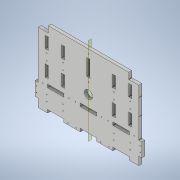
# Autodesk Inventor part: Side_one
Saved by Autodesk Inventor 2020 (Build 240168000, 168)
## iProperties
Created: 2019-12-17
Part Number: Side_one
Material: Generic
Document SubType Name: Modeling
Designer: fabfarm
Density: 1 g/cm^3
Appearance: Default
Author: fabfarm
Autodesk Inventor part; units mm, degrees
ref_plane "YZ Plane" through (0, 0, 0) normal (1, 0, 0) x (0, 1, 0)
ref_plane "XZ Plane" through (0, 0, 0) normal (0, 1, 0) x (-1, 0, 0)
ref_plane "XY Plane" through (0, 0, 0) normal (0, 0, 1) x (1, 0, 0)
sketch "Sketch1" plane through (0, 0, 0) normal (0, 0, 1) x (1, 0, 0)
  line L0 (0, 0) -> (-652, 0)
  line L1 (-652, 0) -> (-652, 464.3)
  line L2 (-652, 464.3) -> (0, 464.3)
  line L3 (0, 464.3) -> (0, 0)
  dimension "d0" = 464.3
  dimension "d1" = 652
  constraints: 8 end point, 2 parallel, 1 horizontal, 1 perpendicular
  measures "d0" distance of L2.end L0.start
  measures "d1" distance of L0.start L0.end
extrude "Extrusion1" add sketch "Sketch1" along normal blind 18.55
sketch "Sketch2" plane through (0, 0, 18.55) normal (0, 0, 1) x (1, 0, 0)
  line L0 (-652, 464.3) -> (-652, 0) projected
  line L1 (-652, 464.3) -> (-633.45, 464.3)
  line L2 (-633.45, 464.3) -> (-633.45, 359.9)
  line L3 (-633.45, 359.9) -> (-652, 359.9)
  line L4 (-652, 359.9) -> (-652, 464.3)
  line L5 (0, 464.3) -> (-652, 464.3) projected
  line L6 (-652, 259.9) -> (-633.45, 259.9)
  line L7 (-633.45, 259.9) -> (-633.45, 134.8)
  line L8 (-633.45, 134.8) -> (-652, 134.8)
  line L9 (-652, 134.8) -> (-652, 259.9)
  point P0 (-652, 359.9)
  point P1 (-652, 134.8)
  dimension "d54" = 18.55
  dimension "d55" = 104.4
  dimension "d86" = 100
  dimension "d87" = 125.1
  constraints: 16 end point, 4 parallel, 2 collinear, 2 horizontal, 2 perpendicular, 2 point on line
  measures "d54" distance of L1.start L1.end
  measures "d55" distance of L1.end L2.end
  measures "d86" distance between parallel lines of L6 L3
  measures "d87" distance of L6.end L7.end
extrude "Extrusion2" cut sketch "Sketch2" against normal blind 18.55
ref_plane "Work Plane1" through (-326, 259.9, 0) normal (-1, 0, 0) x (0, 0, 1)
mirror "Mirror1" about plane through (-326, 259.9, 0) normal (-1, 0, 0) of "Extrusion2"
sketch "Sketch3" plane through (0, 0, 18.55) normal (0, 0, 1) x (1, 0, 0)
  line L0 (0, 464.3) -> (-652, 464.3) projected
  line L1 (-652, 426.35) -> (-572, 426.35)
  line L2 (-572, 426.35) -> (-572, 464.3)
  line L3 (-572, 464.3) -> (-652, 464.3)
  line L4 (-652, 464.3) -> (-652, 426.35)
  point P0 (0, 0)
  point P1 (-18.55, 350)
  dimension "d19" = 80
  dimension "d22" = 37.95
  constraints: 8 end point, 2 perpendicular, 1 parallel, 2 other
  measures "d19" distance of L3.end L2.end
  measures "d22" distance of L3.end L1.start
extrude "Extrusion3" cut sketch "Sketch3" against normal blind 18.55
mirror "Mirror2" about plane through (-326, 259.9, 0) normal (-1, 0, 0) of "Extrusion3"
sketch "Sketch4" plane through (0, 0, 18.55) normal (0, 0, 1) x (1, 0, 0)
  line L0 (-576, 134.8) -> (-476, 134.8)
  line L1 (-476, 134.8) -> (-476, 153.35)
  line L2 (-476, 153.35) -> (-576, 153.35)
  line L3 (-576, 153.35) -> (-576, 134.8)
  line L4 (-376, 134.8) -> (-276, 134.8)
  line L5 (-276, 134.8) -> (-276, 153.35)
  line L6 (-276, 153.35) -> (-376, 153.35)
  line L7 (-376, 153.35) -> (-376, 134.8)
  line L8 (-176, 134.8) -> (-76, 134.8)
  line L9 (-76, 134.8) -> (-76, 153.35)
  line L10 (-76, 153.35) -> (-176, 153.35)
  line L11 (-176, 153.35) -> (-176, 134.8)
  line L12 (0, 0) -> (0, 359.9) projected
  line L13 (-652, 359.9) -> (-652, 0) projected
  line L14 (-633.45, 134.8) -> (-652, 134.8) projected
  line L15 (-652, 259.9) -> (-633.45, 259.9) projected
  dimension "d59" = 100
  dimension "d60" = 100
  dimension "d61" = 100
  dimension "d62" = 100
  dimension "d63" = 100
  dimension "d66" = 18.55
  dimension "d67" = 76
  constraints: 24 end point, 6 parallel, 5 collinear, 3 horizontal, 3 perpendicular
  measures "d59" distance of L1.end L2.end
  measures "d60" distance of L5.end L6.end
  measures "d61" distance between parallel lines of L1 L7
  measures "d62" distance between parallel lines of L11 L5
  measures "d63" distance of L9.end L10.end
  measures "d66" distance of L2.end L0.start
  measures "d67" distance between parallel lines of L12 L9
extrude "Extrusion4" cut sketch "Sketch4" against normal blind 20
sketch "Sketch6" plane through (0, 0, 18.55) normal (0, 0, 1) x (1, 0, 0)
  line L0 (-276, 400.4) -> (-376, 400.4)
  line L1 (-376, 400.4) -> (-376, 425.4)
  line L2 (-376, 425.4) -> (-276, 425.4)
  line L3 (-276, 425.4) -> (-276, 400.4)
  line L4 (-276, 400.4) -> (-376, 425.4) construction
  line L5 (-376, 400.4) -> (-276, 425.4) construction
  line L6 (-326, -92.86) -> (-326, 557.16) projected
  line L7 (-80, 464.3) -> (-572, 464.3) projected
  point P0 (0, 0)
  point P1 (-326, 412.9)
  dimension "d38" = 25
  dimension "d39" = 100
  dimension "d40" = 38.9
  constraints: 12 end point, 2 midpoint, 2 parallel, 1 horizontal, 1 perpendicular, 1 point on line
  measures "d38" distance of L0.end L1.end
  measures "d39" distance of L1.end L2.end
  measures "d40" distance between parallel lines of L7 L2
extrude "Extrusion6" [suppressed]
fillet "Fillet1" [suppressed]
sketch "Sketch7" plane through (0, 0, 18.55) normal (0, 0, 1) x (1, 0, 0)
  line L0 (-590.55, 183.35) -> (-572, 183.35)
  line L1 (-572, 183.35) -> (-572, 253.85)
  line L2 (-572, 253.85) -> (-590.55, 253.85)
  line L3 (-590.55, 253.85) -> (-590.55, 183.35)
  line L4 (-490.6, 183.35) -> (-472.05, 183.35)
  line L5 (-472.05, 183.35) -> (-472.05, 253.85)
  line L6 (-472.05, 253.85) -> (-490.6, 253.85)
  line L7 (-490.6, 253.85) -> (-490.6, 183.35)
  line L8 (-572, 464.3) -> (-572, 426.35) projected
  line L9 (-576, 153.35) -> (-476, 153.35) projected
  point P0 (0, 0)
  point P1 (-572, 290)
  dimension "d44" = 81.4
  dimension "d45" = 18.55
  dimension "d46" = 70.5
  dimension "d72" = 30
  constraints: 16 end point, 4 parallel, 2 collinear, 2 horizontal, 2 perpendicular, 2 point on line
  measures "d44" distance between parallel lines of L7 L1
  measures "d45" distance of L1.end L2.end
  measures "d46" distance of L2.end L0.start
  measures "d72" distance between parallel lines of L9 L0
extrude "Extrusion7" cut sketch "Sketch7" against normal blind 20
mirror "Mirror3" about plane through (-326, 259.9, 0) normal (-1, 0, 0) of "Extrusion7"
sketch "Esquisse8" plane through (0, 0, 0) normal (0, 0, -1) x (-1, 0, 0)
  line L0 (80, 334.35) -> (61.45, 334.35)
  line L1 (61.45, 334.35) -> (61.45, 404.85)
  line L2 (61.45, 404.85) -> (80, 404.85)
  line L3 (80, 404.85) -> (80, 334.35)
  line L4 (161.4, 404.85) -> (179.95, 404.85)
  line L5 (179.95, 404.85) -> (179.95, 334.35)
  line L6 (179.95, 334.35) -> (161.4, 334.35)
  line L7 (161.4, 334.35) -> (161.4, 404.85)
  line L8 (61.45, 183.35) -> (61.45, 253.85) projected
  line L9 (80, 253.85) -> (80, 183.35) projected
  line L10 (161.4, 183.35) -> (161.4, 253.85) projected
  line L11 (179.95, 253.85) -> (179.95, 183.35) projected
  line L12 (80, 253.85) -> (61.45, 253.85) projected
  point P0 (0, 0)
  dimension "d51" = 70.5
  dimension "d90" = 80.5
  constraints: 16 end point, 4 collinear, 4 parallel, 2 horizontal, 2 perpendicular, 2 point on line
  measures "d51" distance of L0.end L1.end
  measures "d90" distance between parallel lines of L0 L12
extrude "Extrusion8" cut sketch "Esquisse8" against normal blind 20
mirror "Symétrie4" about plane through (-326, 259.9, 0) normal (-1, 0, 0) of "Extrusion8"
sketch "Esquisse9" plane through (0, 0, 18.55) normal (0, 0, 1) x (1, 0, 0)
  circle A0 centre (-634.5708, 361.0208) radius 1.585
  circle A1 centre (-634.5708, 135.9208) radius 1.585
  circle A2 centre (-589.4292, 403.7292) radius 1.585
  circle A3 centre (-589.4292, 335.4708) radius 1.585
  circle A4 centre (-634.5708, 258.7792) radius 1.585
  circle A5 centre (-589.4292, 252.7292) radius 1.585
  circle A6 centre (-573.1208, 252.7292) radius 1.585
  circle A7 centre (-573.1208, 184.4708) radius 1.585
  circle A8 centre (-573.1208, 427.4708) radius 1.585
  circle A9 centre (-574.8792, 152.2292) radius 1.585
  circle A10 centre (-374.8792, 152.2292) radius 1.585
  line L0 (-80, 464.3) -> (-572, 464.3) projected
  line L1 (-326, 464.3) -> (-325.9857, 153.4511) construction
  circle A11 centre (-574.8792, 135.9208) radius 1.585
  circle A12 centre (-374.8792, 135.9208) radius 1.585
  line L2 (-633.45, 359.9) -> (-634.5708, 361.0208) construction
  line L3 (-633.45, 426.35) -> (-633.45, 359.9) projected
  line L4 (-633.45, 259.9) -> (-634.5708, 258.7792) construction
  line L5 (-634.5708, 135.9208) -> (-633.45, 134.8) construction
  line L6 (-633.45, 259.9) -> (-633.45, 134.8) projected
  line L7 (-633.45, 426.35) -> (-572, 426.35) projected
  line L8 (-573.1208, 427.4708) -> (-572, 426.35) construction
  line L9 (-590.55, 404.85) -> (-589.4292, 403.7292) construction
  circle A13 centre (-573.1208, 335.4708) radius 1.585
  line L10 (-573.1208, 335.4708) -> (-572, 334.35) construction
  line L11 (-590.55, 334.35) -> (-589.4292, 335.4708) construction
  line L12 (-572, 334.35) -> (-590.55, 334.35) projected
  line L13 (-573.1208, 184.4708) -> (-572, 183.35) construction
  line L14 (-573.1208, 252.7292) -> (-572, 253.85) construction
  line L15 (-572, 253.85) -> (-572, 183.35) projected
  line L16 (-590.55, 183.35) -> (-589.4292, 184.4708) construction
  line L17 (-572, 183.35) -> (-590.55, 183.35) projected
  circle A14 centre (-589.4292, 184.4708) radius 1.585
  line L18 (-572, 334.35) -> (-572, 464.3) projected
  line L19 (-572, 399.325) -> (-490.6, 369.6) construction
  line L20 (-490.6, 334.35) -> (-490.6, 404.85) construction
  line L21 (-531.3, 384.4625) -> (-531.3, 153.45) construction
  circle A15 centre (-473.1708, 403.7292) radius 1.585
  circle A16 centre (-473.1708, 335.4708) radius 1.585
  circle A17 centre (-473.1708, 252.7292) radius 1.585
  circle A18 centre (-489.4792, 252.7292) radius 1.585
  circle A19 centre (-489.4792, 184.4708) radius 1.585
  line L22 (-472.05, 404.85) -> (-473.1708, 403.7292) construction
  circle A20 centre (-489.4792, 335.4708) radius 1.585
  line L23 (-489.4792, 335.4708) -> (-490.6, 334.35) construction
  line L24 (-472.05, 334.35) -> (-473.1708, 335.4708) construction
  line L25 (-489.4792, 184.4708) -> (-490.6, 183.35) construction
  line L26 (-489.4792, 252.7292) -> (-490.6, 253.85) construction
  line L27 (-472.05, 183.35) -> (-473.1708, 184.4708) construction
  circle A21 centre (-473.1708, 184.4708) radius 1.585
  line L28 (-490.6, 334.35) -> (-490.6, 404.85)
  line L29 (-490.6, 399.325) -> (-572, 369.6) construction
  line L30 (-476, 134.8) -> (-576, 134.8) construction
  line L31 (-574.8792, 135.9208) -> (-576, 134.8) construction
  line L32 (-576, 153.35) -> (-476, 153.35) construction
  line L33 (-526, 153.35) -> (-526, 134.8) construction
  circle A22 centre (-477.1208, 152.2292) radius 1.585
  circle A23 centre (-477.1208, 135.9208) radius 1.585
  circle A24 centre (-17.4198, 361.0491) radius 1.585
  circle A25 centre (-17.3991, 135.9491) radius 1.585
  circle A26 centre (-78.9803, 403.6546) radius 1.585
  line L34 (-62.5652, 403.7534) -> (-78.9803, 403.6546) construction
  circle A27 centre (-62.5652, 403.7534) radius 1.585
  circle A28 centre (-62.5589, 335.4949) radius 1.585
  circle A29 centre (-17.4104, 258.8076) radius 1.585
  circle A30 centre (-62.5513, 252.7534) radius 1.585
  circle A31 centre (-78.8598, 252.7519) radius 1.585
  circle A32 centre (-78.8536, 184.4934) radius 1.585
  circle A33 centre (-78.8759, 427.4934) radius 1.585
  circle A34 centre (-77.0921, 152.2521) radius 1.585
  circle A35 centre (-277.0921, 152.2337) radius 1.585
  circle A36 centre (-77.0906, 135.9436) radius 1.585
  circle A37 centre (-277.0906, 135.9253) radius 1.585
  line L35 (-18.5404, 359.9282) -> (-17.4198, 361.0491) construction
  line L36 (-18.5465, 426.3782) -> (-18.5404, 359.9282)
  line L37 (-18.5312, 259.9282) -> (-17.4104, 258.8076) construction
  line L38 (-17.3991, 135.9491) -> (-18.5198, 134.8282) construction
  line L39 (-18.5312, 259.9282) -> (-18.5198, 134.8282)
  line L40 (-18.5465, 426.3782) -> (-79.9965, 426.3726)
  line L41 (-78.8759, 427.4934) -> (-79.9965, 426.3726) construction
  line L42 (-79.9945, 404.8726) -> (-61.4445, 404.8743)
  line L43 (-61.4445, 404.8743) -> (-62.5652, 403.7534) construction
  line L44 (-79.9945, 404.8726) -> (-78.9803, 403.6546) construction
  circle A38 centre (-78.8674, 335.4934) radius 1.585
  line L45 (-78.8674, 335.4934) -> (-79.9881, 334.3726) construction
  line L46 (-61.4381, 334.3743) -> (-62.5589, 335.4949) construction
  line L47 (-79.9881, 334.3726) -> (-61.4381, 334.3743)
  line L48 (-78.8536, 184.4934) -> (-79.9742, 183.3726) construction
  line L49 (-78.8598, 252.7519) -> (-79.9807, 253.8726) construction
  line L50 (-79.9807, 253.8726) -> (-79.9742, 183.3726)
  line L51 (-61.4242, 183.3743) -> (-62.5451, 184.4949) construction
  line L52 (-79.9742, 183.3726) -> (-61.4242, 183.3743)
  circle A39 centre (-62.5451, 184.4949) radius 1.585
  line L53 (-79.9881, 334.3726) -> (-79.9945, 404.8726)
  line L54 (-79.994, 399.3476) -> (-161.3913, 369.6151) construction
  line L55 (-161.3881, 334.3651) -> (-161.3945, 404.8651) construction
  line L56 (-120.6927, 384.4813) -> (-120.6715, 153.4688) construction
  circle A40 centre (-162.5013, 252.7442) radius 1.585
  circle A41 centre (-162.4951, 184.4858) radius 1.585
  circle A42 centre (-162.1087, 403.6455) radius 1.4133
  circle A43 centre (-178.8098, 252.7427) radius 1.585
  line L57 (-162.4951, 184.4858) -> (-161.3742, 183.3651) construction
  line L58 (-162.5013, 252.7442) -> (-161.3807, 253.8651) construction
  line L59 (-179.9242, 183.3634) -> (-178.8036, 184.4843) construction
  circle A44 centre (-178.8036, 184.4843) radius 1.585
  line L60 (-178.8237, 403.7427) -> (-162.1087, 403.6455) construction
  circle A45 centre (-178.8174, 335.4843) radius 1.585
  line L61 (-179.9381, 334.3634) -> (-178.8174, 335.4843) construction
  circle A46 centre (-162.5089, 335.4858) radius 1.585
  line L62 (-161.394, 399.3401) -> (-79.9913, 369.6226) construction
  line L63 (-161.3881, 334.3651) -> (-161.3945, 404.8651)
  line L64 (-162.5089, 335.4858) -> (-161.3881, 334.3651) construction
  circle A47 centre (-178.8237, 403.7427) radius 1.585
  line L65 (-179.9445, 404.8634) -> (-178.8237, 403.7427) construction
  line L66 (-161.3945, 404.8651) -> (-162.1087, 403.6455) construction
  line L67 (-175.9698, 134.8138) -> (-75.9698, 134.8229) construction
  line L68 (-77.0906, 135.9436) -> (-75.9698, 134.8229) construction
  line L69 (-75.9715, 153.3729) -> (-175.9715, 153.3638) construction
  line L70 (-125.9715, 153.3684) -> (-125.9698, 134.8184) construction
  circle A48 centre (-174.8506, 152.2431) radius 1.585
  circle A49 centre (-174.8491, 135.9346) radius 1.585
  line L71 (-590.55, 404.85) -> (-572, 404.85) projected
  circle A50 centre (-573.1208, 403.7292) radius 1.585
  line L72 (-572, 404.85) -> (-573.1208, 403.7292) construction
  circle A51 centre (-489.4792, 403.7292) radius 1.585
  point P0 (-476, 153.35)
  point P1 (-472.05, 183.35)
  point P2 (-276, 153.35)
  point P3 (-472.05, 404.85)
  point P4 (-376, 134.8)
  point P5 (-175.9715, 153.3638)
  point P6 (-179.9242, 183.3634)
  point P7 (-179.9445, 404.8634)
  point P8 (-75.9715, 153.3729)
  point P9 (-275.9698, 134.8046)
  dimension "d69" = 3.17
  dimension "d115" = 45
  dimension "d117" = 45
  dimension "d118" = 45
  dimension "d119" = 45
  dimension "d123" = 45
  dimension "d129" = 45
  dimension "d130" = 45
  dimension "d131" = 45
  dimension "d132" = 45
  dimension "d143" = 45
  dimension "d144" = 45
  constraints: 120 end point, 86 symmetric about line, 14 coincident, 11 centre point, 6 vertical, 5 horizontal alignment, 5 midpoint, 3 vertical alignment, 159 other
  measures "d115" angle of L3 L2
  measures "d117" angle of L6 L5
  measures "d118" angle of L6 L4
  measures "d119" angle of L7 L8
  measures "d123" angle of L12 L11
  measures "d129" angle of L15 L14
  measures "d130" angle of L15 L13
  measures "d131" angle of L17 L16
  measures "d132" angle of L30 L31
  measures "d143" angle of L9 L71
  measures "d144" angle of L18 L72
extrude "Extrusion9" cut sketch "Esquisse9" against normal blind 20
sketch "Esquisse11" plane through (0, 0, 18.55) normal (0, 0, 1) x (1, 0, 0)
  circle A0 centre (-642.725, 329.9) radius 2.25
  circle A1 centre (-642.725, 289.9) radius 2.25
  circle A2 centre (-581.275, 314.35) radius 2.25
  circle A3 centre (-581.275, 273.85) radius 2.25
  circle A4 centre (-481.325, 314.35) radius 2.25
  circle A5 centre (-481.325, 273.85) radius 2.25
  line L0 (-572, 334.35) -> (-590.55, 334.35) projected
  line L1 (-581.275, 334.35) -> (-581.275, 253.85) construction
  line L2 (-590.55, 253.85) -> (-572, 253.85) projected
  line L3 (-472.05, 334.35) -> (-490.6, 334.35) projected
  line L4 (-481.325, 334.35) -> (-481.325, 253.85) construction
  line L5 (-490.6, 253.85) -> (-472.05, 253.85) projected
  line L6 (-633.45, 359.9) -> (-652, 359.9) projected
  line L7 (-80, 464.3) -> (-572, 464.3) projected
  line L8 (-326, 464.3) -> (-326, 153.35) construction
  line L9 (-376, 153.35) -> (-276, 153.35) projected
  circle A6 centre (-9.275, 329.9) radius 2.25
  circle A7 centre (-9.275, 289.9) radius 2.25
  circle A8 centre (-70.725, 314.35) radius 2.25
  circle A9 centre (-70.725, 273.85) radius 2.25
  circle A10 centre (-170.675, 314.35) radius 2.25
  circle A11 centre (-170.675, 273.85) radius 2.25
  line L10 (-70.725, 334.35) -> (-70.725, 253.85) construction
  line L11 (-63.6915, 253.85) -> (-77.7585, 253.85)
  line L12 (-178.265, 334.65) -> (-162.585, 334.65)
  line L13 (-170.675, 334.35) -> (-170.675, 253.85) construction
  line L14 (-162.585, 253.65) -> (-178.265, 253.65)
  line L15 (-16.3085, 359.9) -> (0, 359.9)
  line L16 (-652, 259.9) -> (-633.45, 259.9) projected
  line L17 (-642.725, 359.9) -> (-642.725, 259.9) construction
  point P0 (-573.5723, 199.8)
  point P1 (-588.3085, 334.35)
  point P2 (-588.3085, 253.85)
  point P3 (-574.2415, 253.85)
  point P4 (-473.735, 334.65)
  point P5 (-489.415, 334.65)
  point P6 (-489.415, 253.65)
  point P7 (-473.735, 253.65)
  point P8 (-635.6915, 359.9)
  point P9 (-373.7585, 153.35)
  point P10 (-277.485, 153.35)
  point P11 (-178.265, 253.65)
  point P12 (-635.6915, 259.9)
  point P13 (-490.6, 334.35)
  dimension "d76" = 4.5
  dimension "d79" = 30
  dimension "d80" = 20
  dimension "d81" = 20
  dimension "d82" = 20
  dimension "d83" = 20
  dimension "d91" = 30
  constraints: 18 symmetric about line, 16 end point, 12 centre point, 10 point on line, 5 equal radius, 5 midpoint, 18 other
  measures "d76" diameter of A0
  measures "d79" distance from line of L6 A0.centre
  measures "d80" distance from line of L2 A3.centre
  measures "d91" distance from line of A1.centre L16
extrude "Extrusion10" cut sketch "Esquisse11" against normal blind 20
sketch "Esquisse12" plane through (0, 0, 18.55) normal (0, 0, 1) x (1, 0, 0)
  line L0 (-652, 0) -> (0, 0) projected
  line L1 (-576, 0) -> (-476, 0)
  line L2 (-476, 0) -> (-476, 18.55)
  line L3 (-476, 18.55) -> (-576, 18.55)
  line L4 (-576, 18.55) -> (-576, 0)
  line L5 (-376, 0) -> (-276, 0)
  line L6 (-276, 0) -> (-276, 18.55)
  line L7 (-276, 18.55) -> (-376, 18.55)
  line L8 (-376, 18.55) -> (-376, 0)
  line L9 (-176, 0) -> (-76, 0)
  line L10 (-76, 0) -> (-76, 18.55)
  line L11 (-76, 18.55) -> (-176, 18.55)
  line L12 (-176, 18.55) -> (-176, 0)
  line L13 (-476, 153.35) -> (-476, 134.8) projected
  line L14 (-576, 134.8) -> (-576, 153.35) projected
  line L15 (-376, 134.8) -> (-376, 153.35) projected
  line L16 (-276, 153.35) -> (-276, 134.8) projected
  line L17 (-176, 134.8) -> (-176, 153.35) projected
  line L18 (-76, 153.35) -> (-76, 134.8) projected
  point P0 (-475.9, 151.865)
  point P1 (-475.9, 136.385)
  point P2 (-576, 137.0415)
  point P3 (-576, 151.1085)
  point P4 (-376, 137.0415)
  point P5 (-376, 151.1085)
  point P6 (-275.9, 151.865)
  point P7 (-275.9, 136.385)
  point P8 (-176.1, 136.385)
  point P9 (-176.1, 151.865)
  point P10 (-75.9, 151.865)
  point P11 (-75.9, 136.385)
  point P12 (-76, 0)
  point P13 (-476, 0)
  point P14 (-276, 0)
  dimension "d92" = 18.55
  constraints: 24 end point, 6 parallel, 4 point on line, 4 vertical, 3 collinear, 3 horizontal, 3 perpendicular, 4 other
  measures "d92" distance of L3.end L1.start
extrude "Extrusion11" cut sketch "Esquisse12" against normal blind 20
sketch "Esquisse13" plane through (0, 0, 18.55) normal (0, 0, 1) x (1, 0, 0)
  circle A0 centre (-574.8686, 17.4186) radius 1.6
  line L0 (-576, 0) -> (-576, 18.55) construction
  line L1 (-576, 18.55) -> (-574.8686, 17.4186) construction
  line L2 (-576, 18.55) -> (-476, 18.55) projected
  circle A1 centre (-477.1314, 17.4186) radius 1.6
  circle A2 centre (-374.8686, 17.4186) radius 1.6
  line L3 (-326, 18.55) -> (-326, 134.8) construction
  line L4 (-276, 134.8) -> (-376, 134.8) projected
  line L5 (-376, 18.55) -> (-276, 18.55) projected
  circle A3 centre (-77.1314, 17.4186) radius 1.6
  line L6 (-76, 0) -> (-76, 18.55) construction
  line L7 (-76, 18.55) -> (-77.1314, 17.4186) construction
  line L8 (-76, 18.55) -> (-176, 18.55) construction
  circle A4 centre (-174.8686, 17.4186) radius 1.6
  circle A5 centre (-277.1314, 17.4186) radius 1.6
  point P0 (0, 0)
  point P1 (-176, 18.55)
  point P2 (-76, 18.55)
  point P3 (-278.2069, 134.8)
  point P4 (-373.7585, 134.8)
  point P5 (-173.7373, 18.55)
  point P6 (-478.2627, 18.55)
  dimension "d95" = 3.2
  dimension "d133" = 45
  constraints: 10 end point, 6 symmetric about line, 4 vertical, 2 horizontal alignment, 2 midpoint, 18 other
  measures "d133" angle of L2 L1
extrude "Extrusion12" cut sketch "Esquisse13" against normal blind 20
sketch "Esquisse14" plane through (0, 0, 18.55) normal (0, 0, 1) x (1, 0, 0)
  circle A0 centre (-581.275, 94.8) radius 2.25
  circle A1 centre (-581.275, 58.55) radius 2.25
  circle A2 centre (-481.325, 94.8) radius 2.25
  circle A3 centre (-481.325, 58.55) radius 2.25
  line L0 (-572, 183.35) -> (-590.55, 183.35) projected
  line L1 (-581.275, 183.35) -> (-581.275, 0) construction
  line L2 (-652, 0) -> (-576, 0) projected
  line L3 (-472.05, 183.35) -> (-490.6, 183.35) projected
  line L4 (-481.325, 183.35) -> (-481.325, -0.1) construction
  line L5 (-573.7373, 18.55) -> (-476, 18.55) projected
  line L6 (-476, 134.8) -> (-576, 134.8) projected
  line L7 (-376, 18.55) -> (-276, 18.55) projected
  line L8 (-326, 18.55) -> (-326, 134.8) construction
  line L9 (-276, 134.8) -> (-376, 134.8) projected
  circle A4 centre (-70.725, 94.8) radius 2.25
  circle A5 centre (-70.725, 58.55) radius 2.25
  circle A6 centre (-170.675, 94.8) radius 2.25
  circle A7 centre (-170.675, 58.55) radius 2.25
  point P0 (0, 0)
  point P1 (-477.5, 18.55)
  point P2 (-477.485, 134.8)
  point P3 (-573.7585, 134.8)
  point P4 (-374.5, 18.55)
  point P5 (-277.5, 18.55)
  point P6 (-277.485, 134.8)
  point P7 (-373.7585, 134.8)
  dimension "d98" = 4.5
  dimension "d99" = 40
  dimension "d100" = 40
  dimension "d101" = 40
  dimension "d103" = 40
  constraints: 8 centre point, 6 end point, 5 point on line, 4 midpoint, 4 symmetric about line, 3 equal radius, 2 vertical, 4 other
  measures "d98" diameter of A0
  measures "d99" distance from line of L5 A3.centre
  measures "d100" distance from line of L6 A2.centre
  measures "d101" distance from line of L6 A0.centre
  measures "d103" distance from line of L5 A1.centre
extrude "Extrusion13" cut sketch "Esquisse14" against normal blind 20
sketch "Esquisse16" plane through (0, 0, 18.55) normal (0, 0, 1) x (1, 0, 0)
  line L0 (0, 0) -> (0, 134.8) projected
  line L1 (-76, 0) -> (0, 0) projected
  line L2 (0, 50) -> (-18.55, 50)
  line L3 (-18.55, 50) -> (-18.55, 0)
  line L4 (-18.55, 0) -> (0, 0)
  line L5 (0, 0) -> (0, 50)
  line L6 (-18.55, 134.8) -> (-18.55, 259.9) projected
  line L7 (0, 134.8) -> (-18.55, 134.8) projected
  line L8 (-652, 0) -> (-576, 0) projected
  line L9 (-652, 50) -> (-633.45, 50)
  line L10 (-633.45, 50) -> (-633.45, 0)
  line L11 (-633.45, 0) -> (-652, 0)
  line L12 (-652, 0) -> (-652, 50)
  line L13 (-633.45, 259.9) -> (-633.45, 134.8) projected
  line L14 (-652, 134.8) -> (-652, 0) projected
  point P0 (-18.55, 136.385)
  point P1 (-18.55, 258.315)
  point P2 (-16.965, 134.8)
  dimension "d110" = 50
  dimension "d111" = 84.8
  constraints: 16 end point, 4 collinear, 4 parallel, 3 point on line, 2 horizontal, 2 perpendicular
  measures "d110" distance of L2.end L3.end
  measures "d111" distance between parallel lines of L7 L2
extrude "Extrusion15" cut sketch "Esquisse16" against normal blind 60
sketch "Esquisse18" plane through (0, 0, 18.55) normal (0, 0, 1) x (1, 0, 0)
  line L0 (-633.45, 50) -> (-633.45, 0) projected
  circle A0 centre (-634.5814, 48.8686) radius 1.6
  circle A1 centre (-17.4186, 48.8686) radius 1.6
  line L1 (-18.55, 50) -> (0, 50) construction
  line L2 (-18.55, 50) -> (-17.4186, 48.8686) construction
  line L3 (-18.55, 0) -> (-18.55, 50) construction
  point P0 (0, 0)
  dimension "d136" = 3.2
  dimension "d135" = 45
  constraints: 2 end point, 1 horizontal alignment, 6 other
  measures "d135" angle of L3 L2
extrude "Extrusion16" cut sketch "Esquisse18" against normal blind 20
sketch "Esquisse17" plane through (0, 0, 18.55) normal (0, 0, 1) x (1, 0, 0)
  circle A0 centre (-8.9415, 109.8) radius 2.25
  circle A1 centre (-8.9415, 75) radius 2.25
  circle A2 centre (-643.5228, 109.8) radius 2.25
  circle A3 centre (-643.5228, 75) radius 2.25
  line L0 (-652, 134.8) -> (-633.45, 134.8) projected
  line L1 (-642.725, 134.8) -> (-643.8564, 50) construction
  line L2 (-635.7127, 50) -> (-652, 50) projected
  line L3 (-18.55, 134.8) -> (0, 134.8) construction
  line L4 (-9.275, 134.8) -> (-8.1436, 50) construction
  line L5 (-16.2873, 50) -> (0, 50) construction
  point P0 (0, 0)
  point P1 (-635.6915, 134.8)
  point P2 (-16.3074, 134.8)
  dimension "d134" = 4.5
  dimension "d139" = 25
  dimension "d140" = 25
  constraints: 4 centre point, 4 end point, 4 midpoint, 3 equal radius, 2 horizontal alignment, 2 point on line, 2 vertical alignment
  measures "d134" diameter of A2
  measures "d139" distance from line of L0 A2.centre
  measures "d140" distance from line of A3.centre L2
extrude "Extrusion17" cut sketch "Esquisse17" against normal blind 20
sketch "Esquisse19" plane through (0, 0, 18.55) normal (0, 0, 1) x (1, 0, 0)
  line L0 (-472.05, 402.6085) -> (-472.05, 336.5915) projected
  line L1 (-316.725, 314.3) -> (-335.275, 314.3)
  line L2 (-335.275, 314.3) -> (-335.275, 414.3)
  line L3 (-335.275, 414.3) -> (-316.725, 414.3)
  line L4 (-316.725, 414.3) -> (-316.725, 314.3)
  line L5 (-80, 464.3) -> (-572, 464.3) projected
  line L6 (-326, 464.3) -> (-326, 414.3) construction
  point P0 (0, 0)
  dimension "d169" = 100
  dimension "d170" = 18.55
  dimension "d171" = 50
  constraints: 10 end point, 2 midpoint, 2 parallel, 1 horizontal, 1 perpendicular, 1 vertical
  measures "d169" distance of L3.end L1.start
  measures "d170" distance of L1.start L1.end
  measures "d171" distance between parallel lines of L5 L3
extrude "Extrusion18" cut sketch "Esquisse19" against normal blind 18.55
sketch "Esquisse20" plane through (0, 0, 18.55) normal (0, 0, 1) x (1, 0, 0)
  line L0 (0, 259.9) -> (-18.55, 259.9)
  line L1 (-18.55, 259.9) -> (-18.55, 359.9)
  line L2 (-18.55, 359.9) -> (0, 359.9)
  line L3 (0, 359.9) -> (0, 259.9)
  line L4 (-633.45, 137.0415) -> (-633.45, 257.6585) projected
  line L5 (-633.45, 259.9) -> (-652, 259.9)
  line L6 (-652, 259.9) -> (-652, 359.9)
  line L7 (-652, 359.9) -> (-633.45, 359.9)
  line L8 (-633.45, 359.9) -> (-633.45, 259.9)
  line L9 (0, 359.9) -> (-16.328, 359.9) projected
  line L10 (-652, 359.9) -> (-652, 259.9) projected
  line L11 (-18.55, 362.1603) -> (-18.55, 426.35) projected
  point P0 (0, 0)
  constraints: 16 end point, 5 collinear, 4 parallel, 2 horizontal, 2 perpendicular, 1 point on line
extrude "Extrusion19" cut sketch "Esquisse20" against normal blind 18.55
sketch "Esquisse21" plane through (0, 0, 18.55) normal (0, 0, 1) x (1, 0, 0)
  circle A0 centre (-325.9879, 223.35) radius 25
  line L0 (-325.9879, 223.35) -> (-325.9879, 153.35) construction
  line L1 (-278.2174, 153.35) -> (-373.7585, 153.35) projected
  point P0 (0, 0)
  dimension "d157" = 50
  dimension "d158" = 70
  constraints: 2 end point, 1 centre point, 1 midpoint, 1 vertical
  measures "d157" diameter of A0
  measures "d158" distance of L0.start L0.end
extrude "Extrusion20" cut sketch "Esquisse21" against normal blind 18.55
sketch "Esquisse22" plane through (0, 0, 18.55) normal (0, 0, 1) x (1, 0, 0)
  circle A0 centre (-251, 9) radius 2.25
  circle A1 centre (-201, 9) radius 2.25
  circle A2 centre (-451, 9) radius 2.25
  circle A3 centre (-401, 9) radius 2.25
  line L0 (-476, 16.2873) -> (-476, 0) projected
  line L1 (-376, 0) -> (-376, 16.2873) projected
  line L2 (-276, 16.2873) -> (-276, 0) projected
  line L3 (-176, 0) -> (-176, 16.2873) projected
  line L4 (-276, 0) -> (-176, 0) projected
  point P0 (0, 0)
  dimension "d161" = 25
  dimension "d162" = 25
  dimension "d163" = 25
  dimension "d164" = 25
  dimension "d165" = 4.5
  dimension "d166" = 9
  constraints: 4 centre point, 3 equal radius, 3 horizontal alignment
  measures "d161" distance from line of L0 A2.centre
  measures "d162" distance from line of L1 A3.centre
  measures "d163" distance from line of L2 A0.centre
  measures "d164" distance from line of L3 A1.centre
  measures "d165" diameter of A0
  measures "d166" distance from line of L4 A0.centre
extrude "Extrusion21" cut sketch "Esquisse22" against normal blind 20
sketch "Esquisse24" plane through (0, 0, 18.55) normal (0, 0, 1) x (1, 0, 0)
  circle A0 centre (-334.1436, 413.1686) radius 1.6
  circle A1 centre (-317.8564, 413.1686) radius 1.6
  circle A2 centre (-334.1436, 315.4314) radius 1.6
  line L0 (-316.725, 414.3) -> (-316.725, 314.3) projected
  circle A3 centre (-317.8564, 315.4314) radius 1.6
  line L1 (-335.275, 314.3) -> (-335.275, 414.3) projected
  line L2 (-335.275, 414.3) -> (-334.1436, 413.1686) construction
  circle A4 centre (-326, 289.3) radius 2.25
  line L3 (-335.275, 314.3) -> (-316.725, 314.3) projected
  line L4 (-326, 314.3) -> (-326, 289.3) construction
  circle A5 centre (-325.95, 439.3) radius 2.25
  line L5 (-335.275, 414.3) -> (-316.725, 414.3) projected
  point P0 (0, 0)
  dimension "d173" = 3.2
  dimension "d174" = 45
  dimension "d175" = 4.5
  dimension "d176" = 25
  dimension "d177" = 25
  dimension "d178" = 4.5
  dimension "d179" = 9.325
  constraints: 4 end point, 3 centre point, 2 horizontal alignment, 2 vertical alignment, 1 midpoint, 1 vertical, 12 other
  measures "d174" angle of L1 L2
  measures "d175" diameter of A4
  measures "d176" distance of L4.start L4.end
  measures "d177" distance from line of L5 A5.centre
  measures "d178" diameter of A5
  measures "d179" distance from line of L1 A5.centre
extrude "Extrusion22" cut sketch "Esquisse24" against normal blind 18.55 contours A0 L1 L5 | L5 A0 | A0 L1 | L5 L0 A1 | A1 L5 | L1 A2 | A2 L3 L1 | A1 L0 | L3 A2 | A3 L0 | L0 L3 A3 | A3 L3 | A4 | A5
sketch "Esquisse25" plane through (0, 0, 18.55) normal (0, 0, 1) x (1, 0, 0)
  line L0 (-476, 151.1085) -> (-476, 137.0415) projected
  line L1 (-476, 144.075) -> (-376, 144.075) construction
  line L2 (-376, 137.0415) -> (-376, 151.1085) projected
  circle A0 centre (-446, 144.075) radius 2.25
  circle A1 centre (-406, 144.075) radius 2.25
  circle A2 centre (-246, 144.075) radius 2.25
  circle A3 centre (-206, 144.075) radius 2.25
  circle A4 centre (-46, 144.075) radius 2.25
  circle A5 centre (-606, 144.075) radius 2.25
  line L3 (-576, 137.0415) -> (-576, 151.1085) projected
  line L4 (-76, 153.35) -> (-76, 134.8) projected
  line L5 (-176, 137.0244) -> (-176, 151.1517) projected
  line L6 (-276, 153.35) -> (-276, 134.8) projected
  point P0 (0, 0)
  point P1 (-76, 151.1034)
  point P2 (-76, 137.0937)
  point P3 (-276, 151.085)
  point P4 (-276, 137.0754)
  dimension "d182" = 30
  dimension "d183" = 30
  dimension "d184" = 30
  dimension "d185" = 30
  dimension "d186" = 30
  dimension "d187" = 30
  dimension "d188" = 4.5
  constraints: 6 centre point, 5 equal radius, 5 horizontal alignment, 2 end point, 2 midpoint, 2 point on line, 1 horizontal
  measures "d182" distance from line of L3 A5.centre
  measures "d183" distance from line of L4 A4.centre
  measures "d184" distance from line of L5 A3.centre
  measures "d185" distance from line of L6 A2.centre
  measures "d186" horizontal distance of L2.start A1.centre
  measures "d187" distance from line of L0 A0.centre
  measures "d188" diameter of A1
extrude "Extrusion23" cut sketch "Esquisse25" against normal blind 30
body "Solid1"
